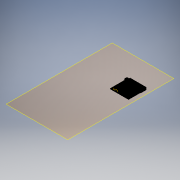
# Autodesk Inventor part: SD_Center
Saved by Autodesk Inventor 2017 SP1 (Build 210196100, 196)
## iProperties
Created: 2016-08-29
Part Number: SD_Center
Material: Generic
Document SubType Name: Modeling
Designer: jwrjc
Density: 1 g/cm^3
Appearance: Default
Author: jwrjc
Autodesk Inventor part; units mm, degrees
ref_plane "YZ Plane" through (0, 0, 0) normal (1, 0, 0) x (0, 1, 0)
ref_plane "XZ Plane" through (0, 0, 0) normal (0, 1, 0) x (-1, 0, 0)
ref_plane "XY Plane" through (0, 0, 0) normal (0, 0, 1) x (1, 0, 0)
sketch "Sketch1" plane through (0, 0, 0) normal (0, 0, 1) x (1, 0, 0)
  line L0 (20.713, 22.6136) -> (8.1882, 22.6136)
  line L1 (8.1882, 22.6136) -> (8.1882, 21.836)
  line L2 (8.1882, 21.836) -> (6.522, 21.836)
  line L3 (6.522, 21.836) -> (6.522, 9.2001)
  line L4 (6.522, 9.2001) -> (20.3798, 9.2001)
  line L5 (20.3798, 9.2001) -> (20.3798, 17.6981)
  line L6 (20.3798, 17.6981) -> (20.713, 18.8367)
  line L7 (20.713, 18.8367) -> (20.713, 22.6136)
  point P0 (0, 0)
  constraints: 16 end point, 5 perpendicular, 1 horizontal, 1 parallel
extrude "Extrusion1" add sketch "Sketch1" along normal blind 0.8
sketch "Sketch2" plane through (0, 0, 0.8) normal (0, 0, 1) x (1, 0, 0)
  line L0 (20.713, 22.6136) -> (8.1882, 22.6136) projected
  line L1 (20.713, 22.6136) -> (20.713, 19.8609)
  line L2 (20.713, 18.8367) -> (20.713, 22.6136) projected
  line L3 (20.713, 19.8609) -> (6.522, 19.8609)
  line L4 (6.522, 21.836) -> (6.522, 9.2001) projected
  line L5 (6.522, 19.8609) -> (6.522, 21.836)
  line L6 (8.1882, 21.836) -> (6.522, 21.836) projected
  line L7 (6.522, 21.836) -> (8.1882, 21.836)
  line L8 (8.1882, 22.6136) -> (8.1882, 21.836) projected
  line L9 (8.1882, 21.836) -> (8.1882, 22.6136)
  line L10 (8.1882, 22.6136) -> (20.713, 22.6136)
  line L11 (20.713, 19.8609) -> (6.522, 19.8609)
  point P0 (0, 0)
  constraints: 14 end point, 2 collinear, 2 perpendicular, 2 point on line, 1 horizontal, 1 vertical
extrude "Extrusion2" add sketch "Sketch2" along normal blind 1
ref_plane "Work Plane1" through (0, 0, 0) normal (0, 0, 1) x (1, 0, 0)
sketch "Sketch3" plane through (0, 0, 0) normal (0, 0, 1) x (1, 0, 0)
  line L0 (6.522, 21.836) -> (6.522, 9.2001) projected
  line L1 (6.0995, 18.511) -> (6.522, 18.511)
  line L2 (6.522, 18.511) -> (6.522, 17.9361)
  line L3 (6.522, 17.9361) -> (6.0995, 17.9361)
  line L4 (6.0995, 17.9361) -> (6.0995, 18.511)
  line L5 (6.0995, 17.5361) -> (6.522, 17.5361)
  line L6 (6.522, 17.5361) -> (6.522, 16.9111)
  line L7 (6.522, 16.9111) -> (6.0995, 16.9111)
  line L8 (6.0995, 16.9111) -> (6.0995, 17.5361)
  line L9 (6.0995, 16.4362) -> (6.522, 16.4362)
  line L10 (6.522, 16.4362) -> (6.522, 15.7862)
  line L11 (6.522, 15.7862) -> (6.0995, 15.7862)
  line L12 (6.0995, 15.7862) -> (6.0995, 16.4362)
  line L13 (6.0995, 15.3613) -> (6.522, 15.3613)
  line L14 (6.522, 15.3613) -> (6.522, 14.8113)
  line L15 (6.522, 14.8113) -> (6.0995, 14.8113)
  line L16 (6.0995, 14.8113) -> (6.0995, 15.3613)
  line L17 (6.0995, 14.2614) -> (6.522, 14.2614)
  line L18 (6.522, 14.2614) -> (6.522, 13.7114)
  line L19 (6.522, 13.7114) -> (6.0995, 13.7114)
  line L20 (6.0995, 13.7114) -> (6.0995, 14.2614)
  line L21 (6.0995, 13.2364) -> (6.522, 13.2364)
  line L22 (6.522, 13.2364) -> (6.522, 12.5365)
  line L23 (6.522, 12.5365) -> (6.0995, 12.5365)
  line L24 (6.0995, 12.5365) -> (6.0995, 13.2364)
  line L25 (6.0995, 12.0365) -> (6.522, 12.0365)
  line L26 (6.522, 12.0365) -> (6.522, 11.4116)
  line L27 (6.522, 11.4116) -> (6.0995, 11.4116)
  line L28 (6.0995, 11.4116) -> (6.0995, 12.0365)
  line L29 (6.0995, 11.0116) -> (6.522, 11.0116)
  line L30 (6.522, 11.0116) -> (6.522, 10.3117)
  line L31 (6.522, 10.3117) -> (6.0995, 10.3117)
  line L32 (6.0995, 10.3117) -> (6.0995, 11.0116)
  line L33 (6.0995, 9.8867) -> (6.522, 9.8867)
  line L34 (6.522, 9.8867) -> (6.522, 9.3367)
  line L35 (6.522, 9.3367) -> (6.0995, 9.3367)
  line L36 (6.0995, 9.3367) -> (6.0995, 9.8867)
  point P0 (0, 0)
  constraints: 72 end point, 18 parallel, 9 horizontal, 9 perpendicular, 7 point on line, 10 other
extrude "Extrusion3" add sketch "Sketch3" along normal blind 0.4 separate body
sketch "Sketch4" plane through (0, 0, 0.8) normal (0, 0, 1) x (1, 0, 0)
  line L0 (20.3798, 9.2001) -> (20.3798, 17.6981) projected
  line L1 (20.3798, 9.2001) -> (12.4, 9.2001)
  line L2 (12.4, 9.2001) -> (12.4, 9.5625)
  line L3 (12.4, 9.5625) -> (20.3798, 9.5625)
  line L4 (20.3798, 9.5625) -> (20.3798, 9.2001)
  point P0 (0, 0)
  constraints: 8 end point, 2 parallel, 1 horizontal, 1 perpendicular
extrude "Extrusion4" add sketch "Sketch4" along normal blind 1 bodies 1
sketch "Sketch5" plane through (0, 0, 0.8) normal (0, 0, 1) x (1, 0, 0)
  line L0 (8.354, 9.3798) -> (9.142, 9.3798)
  line L1 (9.142, 9.3798) -> (10.0366, 10.1915)
  line L2 (10.0366, 10.1915) -> (10.3613, 10.1915)
  line L3 (10.3613, 10.1915) -> (11.3502, 9.6012)
  line L4 (11.3502, 9.6012) -> (12.1472, 9.6012)
  line L5 (12.1472, 9.6012) -> (12.1472, 9.3798)
  line L6 (12.1472, 9.3798) -> (11.3314, 9.3798)
  line L7 (11.3314, 9.3798) -> (10.386, 9.9442)
  line L8 (10.386, 9.9442) -> (10.0513, 9.9442)
  line L9 (10.0513, 9.9442) -> (9.2543, 9.2209)
  line L10 (9.2543, 9.2209) -> (8.354, 9.2209)
  line L11 (8.354, 9.2209) -> (8.354, 9.3798)
  point P0 (0, 0)
  constraints: 24 end point, 6 parallel, 2 perpendicular, 2 point on line, 1 horizontal
extrude "Extrusion5" add sketch "Sketch5" along normal blind 0.75 separate body
fillet "Fillet1" radius 0.05 2 edges at (8.354, 9.2209, 1.175) (8.354, 9.3798, 1.175)
fillet "Fillet2" radius 0.2 8 edges at (10.386, 9.9442, 1.175) (10.0513, 9.9442, 1.175) (9.2543, 9.2209, 1.175) (9.142, 9.3798, 1.175) (10.0366, 10.1915, 1.175) (10.3613, 10.1915, 1.175) (11.3502, 9.6012, 1.175) (11.3314, 9.3798, 1.175)
body "Solid1"
body "Solid2"
body "Solid3"
